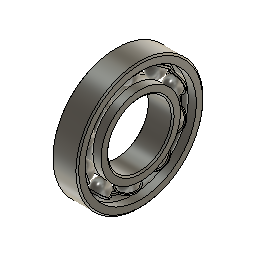
Mechanical_Ball_Bearing (Autodesk Fusion 360 design; units mm, degrees)
part number: 2025-04-03-10-29-34-634
Autodesk Fusion 360 part; units mm, degrees
note: some values were not read from the file. Set by a fixed rule: which face or edge a step refers to.
sketch "Sketch1" plane through (0, 0, 0) normal (0, 1, 0) x (1, 0, 0)
  line L0 (0, 0) -> (100, 0)
  line L1 (-5, -10) -> (5, -10)
  line L2 (5, -10) -> (5, -20)
  line L3 (5, -20) -> (-5, -20)
  line L4 (-5, -20) -> (-5, -10)
  circle A0 centre (0, -15) radius 3.1
  line L5 (-5, -17.5) -> (-1.833, -17.5)
  line L6 (1.833, -17.5) -> (5, -17.5)
  line L7 (0, 0) -> (0, -18)
  line L8 (-5, -12.5) -> (-1.833, -12.5)
  line L9 (1.833, -12.5) -> (5, -12.5)
  circle A1 centre (0, -15) radius 3
  line L10 (-5, -15) -> (2, -15) construction
  line L11 (0, -18) -> (0, -12) construction
  line L12 (0, -18) -> (0, -12)
  dimension "d1" = 20
  dimension "d2" = 40
  dimension "d3" = 10
  dimension "d4" = 2.5
  dimension "d5" = 2.5
  dimension "d6" = 0.1
  dimension "d7" = 6
  dimension "d8" = 5
  constraint coincident L0.start L7.start
  constraint horizontal L0
  constraint horizontal L1
  constraint vertical L2
  constraint horizontal L3
  constraint vertical L4
  constraint perpendicular L3 L7
  constraint symmetric L2 L4 L7
  constraint coincident A0.centre L7
  constraint coincident L4 L5.start
  constraint coincident L2 L6.end
  constraint perpendicular L2 L5
  constraint coincident L4 L8.start
  constraint coincident L2 L9.end
  constraint perpendicular L2 L8
  constraint coincident A0 L5.end
  constraint collinear L5 L6
  constraint coincident A0 L6.start
  constraint coincident A0 L9.start
  constraint collinear L8 L9
  constraint coincident A0 L8.end
  constraint midpoint L4 L10.start
  constraint perpendicular L7 L10
  constraint coincident A0.centre A1.centre
  constraint coincident A1 L11.end
  constraint coincident L7 L11.end
  measures "d3" distance of L2 L4
  measures "d4" distance of L3 L5
  measures "d5" distance of L1 L8
  measures "d6" distance of A0 A1
  measures "d7" diameter of A1
  measures "d8" distance of L3 A0.centre
revolve "Revolve1" add sketch "Sketch1" angle 360 about axis through (0, 0, 0) along (1, 0, 0) contours L1 L4 A0 L7 L8 | L1 L2 A0 L7 L9 makes body 1
revolve "Revolve2" add sketch "Sketch1" angle 360 about axis through (0, 0, 0) along (1, 0, 0) separate body contours L2 L3 L4 A0 L5 L6 makes body 2
revolve "Revolve3" add sketch "Sketch1" angle 360 about axis through (0, 0, 0) along (0, 0, 1) separate body contours L7 A1 L12 picked at (1.9264, -15.3461) makes body 3
pattern_circular "C-Pattern1" count 10 over 360 about axis through (1.75, 0, 0) along (1, 0, 0) of bodies 3 makes body 4 at (1.4872, -10.6705, 10.3044) makes body 5 at (-1.4872, -14.6894, 2.0645) makes body 6 at (-1.4872, -13.0975, -6.964) makes body 7 at (1.4872, -10.6705, -10.3044) makes body 8 at (1.4872, -2.5758, -14.6084) makes body 9 at (1.4872, 10.6705, -10.3044) makes body 10 at (-1.4872, 14.6894, -2.0645) makes body 11 at (1.4872, 13.0975, 6.964) makes body 12 at (1.4872, 6.5027, 13.3325)
chamfer "Chamfer1" distance 0.5 angle 45 2 edges at (5, -3.6162, -9.3233) (-5, -3.6162, -9.3233) on bodies 1
chamfer "Chamfer2" distance 0.5 angle 45 2 edges at (5, -7.2323, -18.6465) (-5, -7.2323, -18.6465) on bodies 2
sketch "Sketch2" plane through (0, 0, 0) normal (1, 0, 0) x (0, 1, 0)
  circle A0 centre (0, 0) radius 16.5
  circle A1 centre (0, 0) radius 16
  dimension "d16" = 33
  dimension "d17" = 32
  constraint coincident A0.centre A1.centre
  constraint concentric A0 A1
  measures "d16" diameter of A0
  measures "d17" diameter of A1
extrude "Extrude1" add sketch "Sketch2" along normal up to surface (5 mm away) separate body makes body 13
combine "Combine1" operation cut target body 13 tool bodies 10 11 12 3 4 5 6 7 8 9 keep tools
move_face "OffsetFaces1" offset -0.1 10 faces at (2.7316, -15.5011, 4.7478) (2.7313, -9.7527, 12.9502) (2.7316, -15.3313, -5.2703) (2.7313, -9.3026, -13.2772) (2.7319, 0.2714, -16.2096) (2.7313, 9.7527, -12.9502) (2.7316, 15.5011, -4.7478) (2.7316, 15.3313, 5.2703) (2.7313, 9.3026, 13.2772) (2.7319, -0.2714, 16.2096) on bodies 13
shell "Shell1" thickness 0.5 removed faces 3 at (3.3333, 4.6939, 15.8183) at (5, 16.2719, -0.8197) at (2.1082, 15.9813, 0.7728) on bodies 13
mirror "Mirror1" about plane through (0, 0, 0) normal (1, 0, 0) of bodies 13 merged
scale "Scale1" factors (0.8, 1, 1) about (-4.5, 0, 20) bodies 2 1 3 4 5 6 7 8 9 10 11 12 13
